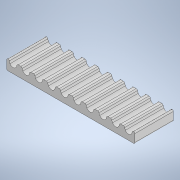
# Autodesk Inventor part: belttunagi
Saved by Autodesk Inventor 2021 (Build 250183000, 183)
## iProperties
Created: 2022-02-13
Part Number: belttunagi
Material: 一般
Document SubType Name: Modeling
Designer: hirohumi
Density: 1 g/cm^3
Appearance: 既定
Author: hirohumi
Autodesk Inventor part; units mm, degrees
ref_plane "YZ Plane" through (0, 0, 0) normal (1, 0, 0) x (0, 1, 0)
ref_plane "XZ Plane" through (0, 0, 0) normal (0, 1, 0) x (-1, 0, 0)
ref_plane "XY Plane" through (0, 0, 0) normal (0, 0, 1) x (1, 0, 0)
sketch "スケッチ1" plane through (0, 0, 0) normal (0, 0, 1) x (1, 0, 0)
  line L0 (-2.5, 0) -> (47.5, 0)
  arc A0 (-1.2061, 2.7902) -> (1.2061, 2.7902) centre (0, 3.44) ccw
  arc A1 (-1.4749, 3.5744) -> (-1.2061, 2.7902) centre (1.03, 3.995) ccw
  arc A2 (1.2061, 2.7902) -> (1.4749, 3.5744) centre (-1.03, 3.995) ccw
  arc A3 (-1.4749, 3.5744) -> (-1.9779, 4) centre (-1.9779, 3.49) ccw
  arc A4 (1.9779, 4) -> (1.4749, 3.5744) centre (1.9779, 3.49) ccw
  line L1 (1.9779, 4) -> (2.5, 4)
  line L2 (-1.9779, 4) -> (-2.5, 4)
  line L3 (6.9779, 4) -> (7.5, 4)
  arc A5 (6.9779, 4) -> (6.4749, 3.5744) centre (6.9779, 3.49) ccw
  arc A6 (6.2061, 2.7902) -> (6.4749, 3.5744) centre (3.97, 3.995) ccw
  arc A7 (3.7939, 2.7902) -> (6.2061, 2.7902) centre (5, 3.44) ccw
  arc A8 (3.5251, 3.5744) -> (3.7939, 2.7902) centre (6.03, 3.995) ccw
  arc A9 (3.5251, 3.5744) -> (3.0221, 4) centre (3.0221, 3.49) ccw
  line L4 (3.0221, 4) -> (2.5, 4)
  line L5 (11.9779, 4) -> (12.5, 4)
  arc A10 (11.9779, 4) -> (11.4749, 3.5744) centre (11.9779, 3.49) ccw
  arc A11 (11.2061, 2.7902) -> (11.4749, 3.5744) centre (8.97, 3.995) ccw
  arc A12 (8.7939, 2.7902) -> (11.2061, 2.7902) centre (10, 3.44) ccw
  arc A13 (8.5251, 3.5744) -> (8.7939, 2.7902) centre (11.03, 3.995) ccw
  arc A14 (8.5251, 3.5744) -> (8.0221, 4) centre (8.0221, 3.49) ccw
  line L6 (8.0221, 4) -> (7.5, 4)
  line L7 (16.9779, 4) -> (17.5, 4)
  arc A15 (16.9779, 4) -> (16.4749, 3.5744) centre (16.9779, 3.49) ccw
  arc A16 (16.2061, 2.7902) -> (16.4749, 3.5744) centre (13.97, 3.995) ccw
  arc A17 (13.7939, 2.7902) -> (16.2061, 2.7902) centre (15, 3.44) ccw
  arc A18 (13.5251, 3.5744) -> (13.7939, 2.7902) centre (16.03, 3.995) ccw
  arc A19 (13.5251, 3.5744) -> (13.0221, 4) centre (13.0221, 3.49) ccw
  line L8 (13.0221, 4) -> (12.5, 4)
  line L9 (21.9779, 4) -> (22.5, 4)
  arc A20 (21.9779, 4) -> (21.4749, 3.5744) centre (21.9779, 3.49) ccw
  arc A21 (21.2061, 2.7902) -> (21.4749, 3.5744) centre (18.97, 3.995) ccw
  arc A22 (18.7939, 2.7902) -> (21.2061, 2.7902) centre (20, 3.44) ccw
  arc A23 (18.5251, 3.5744) -> (18.7939, 2.7902) centre (21.03, 3.995) ccw
  arc A24 (18.5251, 3.5744) -> (18.0221, 4) centre (18.0221, 3.49) ccw
  line L10 (18.0221, 4) -> (17.5, 4)
  line L11 (26.9779, 4) -> (27.5, 4)
  arc A25 (26.9779, 4) -> (26.4749, 3.5744) centre (26.9779, 3.49) ccw
  arc A26 (26.2061, 2.7902) -> (26.4749, 3.5744) centre (23.97, 3.995) ccw
  arc A27 (23.7939, 2.7902) -> (26.2061, 2.7902) centre (25, 3.44) ccw
  arc A28 (23.5251, 3.5744) -> (23.7939, 2.7902) centre (26.03, 3.995) ccw
  arc A29 (23.5251, 3.5744) -> (23.0221, 4) centre (23.0221, 3.49) ccw
  line L12 (23.0221, 4) -> (22.5, 4)
  line L13 (31.9779, 4) -> (32.5, 4)
  arc A30 (31.9779, 4) -> (31.4749, 3.5744) centre (31.9779, 3.49) ccw
  arc A31 (31.2061, 2.7902) -> (31.4749, 3.5744) centre (28.97, 3.995) ccw
  arc A32 (28.7939, 2.7902) -> (31.2061, 2.7902) centre (30, 3.44) ccw
  arc A33 (28.5251, 3.5744) -> (28.7939, 2.7902) centre (31.03, 3.995) ccw
  arc A34 (28.5251, 3.5744) -> (28.0221, 4) centre (28.0221, 3.49) ccw
  line L14 (28.0221, 4) -> (27.5, 4)
  line L15 (36.9779, 4) -> (37.5, 4)
  arc A35 (36.9779, 4) -> (36.4749, 3.5744) centre (36.9779, 3.49) ccw
  arc A36 (36.2061, 2.7902) -> (36.4749, 3.5744) centre (33.97, 3.995) ccw
  arc A37 (33.7939, 2.7902) -> (36.2061, 2.7902) centre (35, 3.44) ccw
  arc A38 (33.5251, 3.5744) -> (33.7939, 2.7902) centre (36.03, 3.995) ccw
  arc A39 (33.5251, 3.5744) -> (33.0221, 4) centre (33.0221, 3.49) ccw
  line L16 (33.0221, 4) -> (32.5, 4)
  line L17 (41.9779, 4) -> (42.5, 4)
  arc A40 (41.9779, 4) -> (41.4749, 3.5744) centre (41.9779, 3.49) ccw
  arc A41 (41.2061, 2.7902) -> (41.4749, 3.5744) centre (38.97, 3.995) ccw
  arc A42 (38.7939, 2.7902) -> (41.2061, 2.7902) centre (40, 3.44) ccw
  arc A43 (38.5251, 3.5744) -> (38.7939, 2.7902) centre (41.03, 3.995) ccw
  arc A44 (38.5251, 3.5744) -> (38.0221, 4) centre (38.0221, 3.49) ccw
  line L18 (38.0221, 4) -> (37.5, 4)
  line L19 (46.9779, 4) -> (47.5, 4)
  arc A45 (46.9779, 4) -> (46.4749, 3.5744) centre (46.9779, 3.49) ccw
  arc A46 (46.2061, 2.7902) -> (46.4749, 3.5744) centre (43.97, 3.995) ccw
  arc A47 (43.7939, 2.7902) -> (46.2061, 2.7902) centre (45, 3.44) ccw
  arc A48 (43.5251, 3.5744) -> (43.7939, 2.7902) centre (46.03, 3.995) ccw
  arc A49 (43.5251, 3.5744) -> (43.0221, 4) centre (43.0221, 3.49) ccw
  line L20 (43.0221, 4) -> (42.5, 4)
  line L21 (-2.5, 4) -> (-2.5, 0)
  line L22 (47.5, 4) -> (47.5, 0)
  point P0 (0, 0)
  point P1 (0, 2.07)
  point P2 (5, 2.07)
  point P3 (10, 2.07)
  point P4 (15, 2.07)
  point P5 (20, 2.07)
  point P6 (25, 2.07)
  point P7 (30, 2.07)
  point P8 (35, 2.07)
  point P9 (40, 2.07)
  point P10 (45, 2.07)
  dimension "d0" = 1.37
  dimension "d1" = 2.54
  dimension "d2" = 2.54
  dimension "d3" = 1.03
  dimension "d4" = 1.03
  dimension "d5" = 0.51
  dimension "d6" = 0.51
  dimension "d7" = 1.93
  dimension "d9" = 5
  dimension "d10" = 2.5
  dimension "d11" = 4
  dimension "d14" = 5
  constraints: 101 point on circle, 50 centre point, 46 end point, 6 tangent, 4 horizontal, 2 vertical, 1 collinear, 1 horizontal alignment, 1 point on line, 1 vertical alignment, 188 other
  measures "d0" radius of A0
  measures "d1" radius of A1
  measures "d2" radius of A2
  measures "d3" horizontal distance of point (0, 0) A1.centre
  measures "d4" horizontal distance of point (0, 0) A2.centre
  measures "d5" radius of A3
  measures "d6" radius of A4
  measures "d7" distance from line of L1 point (0, 2.07)
  measures "d9" distance of L1.end L2.end
  measures "d10" horizontal distance of A0.centre L2.end
  measures "d11" distance between parallel lines of L0 L1
  measures "d14" distance of L1.end L3.end
extrude "押し出し1" add sketch "スケッチ1" along normal blind 15
fillet "フィレット1" radius 0.5 4 edges at (47.5, 0, 7.5) (-2.5, 0, 7.5) (-2.5, 4, 7.5) (47.5, 4, 7.5)
